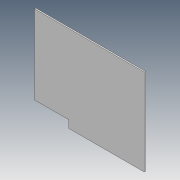
# Autodesk Inventor part: tampa 2
Saved by Autodesk Inventor 2021 (Build 250183000, 183)
## iProperties
Created: 2020-10-21
Part Number: tampa 2
Material: Genérico
Document SubType Name: Modeling
Designer: evert
Density: 1 g/cm^3
Appearance: Padrão
Author: evert
Autodesk Inventor part; units mm, degrees
ref_plane "YZ Plane" through (0, 0, 0) normal (1, 0, 0) x (0, 1, 0)
ref_plane "XZ Plane" through (0, 0, 0) normal (0, 1, 0) x (-1, 0, 0)
ref_plane "XY Plane" through (0, 0, 0) normal (0, 0, 1) x (1, 0, 0)
sketch "Esboço1" plane through (0, 0, 0) normal (0, 0, 1) x (1, 0, 0)
  line L0 (0, 0) -> (50, 0)
  line L1 (50, 0) -> (50, -31.4)
  line L2 (50, -31.4) -> (0, -31.4)
  line L3 (0, -31.4) -> (0, 0)
  dimension "d0" = 50
  dimension "d1" = 31.4
  constraints: 8 end point, 2 parallel, 1 horizontal, 1 perpendicular
  measures "d0" distance of L0.start L0.end
  measures "d1" distance of L2.end L0.start
extrude "Extrusão1" add sketch "Esboço1" along normal blind 0.5
sketch "Esboço2" plane through (0, 0, 0.5) normal (0, 0, 1) x (1, 0, 0)
  line L0 (0, -31.4) -> (50, -31.4) projected
  line L1 (50, -31.4) -> (43.6, -31.4)
  line L2 (43.6, -31.4) -> (43.6, 0)
  line L3 (50, 0) -> (0, 0) projected
  line L4 (43.6, 0) -> (50, 0)
  line L5 (50, -31.4) -> (50, 0) projected
  line L6 (50, 0) -> (50, -31.4)
  dimension "d4" = 6.4
  constraints: 8 end point, 2 point on line, 1 collinear, 1 horizontal, 1 perpendicular
  measures "d4" distance of L0.end L1.end
extrude "Extrusão2" cut sketch "Esboço2" against normal blind 0.5
sketch "Esboço3" plane through (0, 0, 0.5) normal (0, 0, 1) x (1, 0, 0)
  line L0 (0, -31.4) -> (43.6, -31.4) projected
  line L1 (43.6, -31.4) -> (13.6, -31.4)
  line L2 (13.6, -31.4) -> (13.6, -34.4)
  line L3 (13.6, -34.4) -> (43.6, -34.4)
  line L4 (43.6, -34.4) -> (43.6, -31.4)
  point P0 (0, 0)
  dimension "d7" = 30
  dimension "d8" = 3
  constraints: 8 end point, 2 parallel, 1 horizontal, 1 perpendicular
  measures "d7" distance of L3.end L2.end
  measures "d8" distance of L3.end L0.end
extrude "Extrusão3" add sketch "Esboço3" against normal blind 0.5
